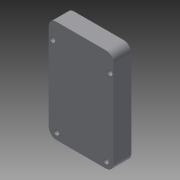
# Autodesk Inventor part: bbb brick
Saved by Autodesk Inventor 2015 (Build 190159000, 159)
## iProperties
Created: 2014-09-09
Part Number: bbb brick
Material: Generic
Document SubType Name: Modeling
Designer: ericd_000
Density: 1 g/cm^3
Appearance: Default
Author: ericd_000
Autodesk Inventor part; units mm, degrees
ref_plane "YZ Plane" through (0, 0, 0) normal (1, 0, 0) x (0, 1, 0)
ref_plane "XZ Plane" through (0, 0, 0) normal (0, 1, 0) x (-1, 0, 0)
ref_plane "XY Plane" through (0, 0, 0) normal (0, 0, 1) x (1, 0, 0)
sketch "Sketch1" plane through (0, 0, 0) normal (0, 1, 0) x (-1, 0, 0)
  line L0 (27.305, 43.18) -> (-27.305, 43.18)
  line L1 (-27.305, 43.18) -> (-27.305, -43.18)
  line L2 (-27.305, -43.18) -> (27.305, -43.18)
  line L3 (27.305, -43.18) -> (27.305, 43.18)
  circle A0 centre (24.265, 28.57) radius 2.225
  circle A1 centre (-24.125, 28.57) radius 2.225
  circle A2 centre (20.955, -37.53) radius 2.225
  circle A3 centre (-20.955, -37.59) radius 2.225
  point P0 (0, 0)
  point P1 (27.305, 0)
  point P2 (0, -43.18)
  dimension "d0" = 86.36
  dimension "d1" = 54.61
  dimension "d2" = 4.45
  dimension "d3" = 4.45
  dimension "d4" = 4.45
  dimension "d5" = 4.45
  dimension "d6" = 48.39
  dimension "d7" = 14.61
  dimension "d8" = 3.18
  dimension "d9" = 41.91
  dimension "d10" = 6.35
  dimension "d11" = 5.59
  dimension "d12" = 66.1
  constraints: 8 end point, 4 centre point, 2 horizontal alignment, 2 midpoint, 2 parallel, 1 horizontal, 1 perpendicular, 1 vertical alignment
  measures "d0" distance of L2.end L0.start
  measures "d1" distance of L1.end L2.end
  measures "d2" diameter of A0
  measures "d3" diameter of A1
  measures "d4" diameter of A3
  measures "d5" diameter of A2
  measures "d6" distance of A1.centre A0.centre
  measures "d7" distance from line of L0 A1.centre
  measures "d8" distance from line of L1 A1.centre
  measures "d9" distance of A2.centre A3.centre
  measures "d10" distance from line of L1 A3.centre
  measures "d11" distance from line of L2 A3.centre
  measures "d12" vertical distance of A2.centre A0.centre
extrude "Extrusion1" add sketch "Sketch1" along normal blind 15
fillet "Fillet1" radius 6.35 4 edges at (-27.305, 7.5, 43.18) (27.305, 7.5, 43.18) (27.305, 7.5, -43.18) (-27.305, 7.5, -43.18)
body "Solid1"
